Autodesk Fusion 360 part; units mm, degrees
(part 5 of 11)
  spline S16 degree 5 poles (47.8745, -68.1891) (47.8941, -68.2177) (47.934, -68.2742) (47.9958, -68.3575) (48.082, -68.4657) (48.1949, -68.5968) (48.3115, -68.7252) (48.4304, -68.8517) (48.5504, -68.9773) (48.6713, -69.1023) (48.793, -69.2265) (48.9159, -69.3498) (49.0402, -69.4719) (49.1663, -69.5925) (49.2941, -69.7117) (49.4235, -69.8295) (49.5542, -69.9462) (49.6861, -70.0619) (49.8189, -70.1767) (49.9526, -70.2907) (50.0871, -70.4039) (50.2227, -70.5162) (50.3592, -70.6276) (50.4968, -70.7381) (50.6354, -70.8476) (50.7749, -70.9562) (50.9154, -71.0639) (51.0567, -71.1709) (51.1988, -71.277) (51.3417, -71.3824) (51.4854, -71.487) (51.6299, -71.5908) (51.7751, -71.6938) (51.9212, -71.796) (52.068, -71.8975) (52.2156, -71.9982) (52.3638, -72.0981) (52.5129, -72.1974) (52.6626, -72.2958) (52.8129, -72.3936) (52.964, -72.4906) (53.1157, -72.587) (53.2681, -72.6826) (53.4212, -72.7775) (53.5749, -72.8717) (53.7292, -72.9652) (53.8842, -73.058) (54.0397, -73.1501) (54.1959, -73.2416) (54.3527, -73.3323) (54.51, -73.4224) (54.668, -73.5118) (54.8265, -73.6006) (54.9856, -73.6887) (55.1453, -73.7761) (55.3055, -73.8629) (55.4663, -73.949) (55.6276, -74.0344) (55.7895, -74.1192) (55.9519, -74.2034) (56.1148, -74.2869) (56.2783, -74.3698) (56.4422, -74.452) (56.6067, -74.5336) (56.7717, -74.6146) (56.9371, -74.695) (57.1031, -74.7747) (57.2696, -74.8537) (57.4365, -74.9322) (57.6039, -75.01) (57.7718, -75.0873) (57.9065, -75.1485) (58.0078, -75.1942) (58.0753, -75.2245) (58.1092, -75.2397) knots 0 0 0 0 0 0 0.01428571 0.02857143 0.04285714 0.05714286 0.07142857 0.08571429 0.1 0.11428571 0.12857143 0.14285714 0.15714286 0.17142857 0.18571429 0.2 0.21428571 0.22857143 0.24285714 0.25714286 0.27142857 0.28571429 0.3 0.31428571 0.32857143 0.34285714 0.35714286 0.37142857 0.38571429 0.4 0.41428571 0.42857143 0.44285714 0.45714286 0.47142857 0.48571429 0.5 0.51428571 0.52857143 0.54285714 0.55714286 0.57142857 0.58571429 0.6 0.61428571 0.62857143 0.64285714 0.65714286 0.67142857 0.68571429 0.7 0.71428571 0.72857143 0.74285714 0.75714286 0.77142857 0.78571429 0.8 0.81428571 0.82857143 0.84285714 0.85714286 0.87142857 0.88571429 0.9 0.91428571 0.92857143 0.94285714 0.95714286 0.97142857 0.98571429 1 1 1 1 1 1
  arc A38 (58.1092, -75.2397) -> (61.7381, -72.3457) centre (0.5538, 0.6546) ccw
  spline S17 degree 5 poles (57.1417, -60.7988) (57.1652, -60.8242) (57.2114, -60.8757) (57.2789, -60.9545) (57.3651, -61.0626) (57.4679, -61.2019) (57.5671, -61.3441) (57.664, -61.4881) (57.7597, -61.6331) (57.8547, -61.7788) (57.9487, -61.9251) (58.0416, -62.0723) (58.1329, -62.2207) (58.2225, -62.3705) (58.3102, -62.5216) (58.3963, -62.6739) (58.481, -62.8274) (58.5644, -62.9817) (58.6468, -63.1367) (58.7282, -63.2924) (58.8086, -63.4488) (58.8879, -63.6059) (58.9662, -63.7638) (59.0432, -63.9225) (59.1192, -64.082) (59.194, -64.2422) (59.2678, -64.4031) (59.3406, -64.5647) (59.4125, -64.7268) (59.4834, -64.8896) (59.5534, -65.053) (59.6224, -65.2169) (59.6905, -65.3815) (59.7577, -65.5466) (59.824, -65.7123) (59.8893, -65.8786) (59.9537, -66.0454) (60.0173, -66.2127) (60.08, -66.3806) (60.1419, -66.549) (60.2029, -66.7178) (60.263, -66.8872) (60.3223, -67.0571) (60.3808, -67.2274) (60.4384, -67.3982) (60.4952, -67.5695) (60.5512, -67.7412) (60.6064, -67.9133) (60.6608, -68.086) (60.7144, -68.259) (60.7673, -68.4325) (60.8193, -68.6064) (60.8705, -68.7807) (60.921, -68.9554) (60.9707, -69.1305) (61.0196, -69.306) (61.0678, -69.4819) (61.1152, -69.6582) (61.1619, -69.8349) (61.2078, -70.0119) (61.253, -70.1894) (61.2974, -70.3672) (61.3411, -70.5453) (61.3841, -70.7238) (61.4263, -70.9027) (61.4678, -71.0819) (61.5086, -71.2614) (61.5486, -71.4413) (61.588, -71.6215) (61.6266, -71.8021) (61.6645, -71.9829) (61.6943, -72.1279) (61.7163, -72.2367) (61.7308, -72.3094) (61.7381, -72.3457) knots 0 0 0 0 0 0 0.01428571 0.02857143 0.04285714 0.05714286 0.07142857 0.08571429 0.1 0.11428571 0.12857143 0.14285714 0.15714286 0.17142857 0.18571429 0.2 0.21428571 0.22857143 0.24285714 0.25714286 0.27142857 0.28571429 0.3 0.31428571 0.32857143 0.34285714 0.35714286 0.37142857 0.38571429 0.4 0.41428571 0.42857143 0.44285714 0.45714286 0.47142857 0.48571429 0.5 0.51428571 0.52857143 0.54285714 0.55714286 0.57142857 0.58571429 0.6 0.61428571 0.62857143 0.64285714 0.65714286 0.67142857 0.68571429 0.7 0.71428571 0.72857143 0.74285714 0.75714286 0.77142857 0.78571429 0.8 0.81428571 0.82857143 0.84285714 0.85714286 0.87142857 0.88571429 0.9 0.91428571 0.92857143 0.94285714 0.95714286 0.97142857 0.98571429 1 1 1 1 1 1
  line L17 (57.1417, -60.7988) -> (56.1297, -59.6994)
  arc A39 (56.1704, -58.5831) -> (56.1297, -59.6994) centre (56.7137, -59.1618) ccw
  arc A40 (56.1704, -58.5831) -> (59.7916, -54.9619) centre (0.5538, 0.6546) ccw
  arc A41 (60.9079, -54.9212) -> (59.7916, -54.9619) centre (60.3703, -55.5052) ccw
  line L18 (60.9079, -54.9212) -> (62.0072, -55.9332)
  spline S18 degree 5 poles (62.0072, -55.9332) (62.0327, -55.9567) (62.0842, -56.003) (62.163, -56.0704) (62.2711, -56.1566) (62.4104, -56.2594) (62.5526, -56.3586) (62.6966, -56.4555) (62.8416, -56.5513) (62.9873, -56.6462) (63.1336, -56.7402) (63.2808, -56.8331) (63.4292, -56.9245) (63.579, -57.014) (63.7301, -57.1018) (63.8824, -57.1878) (64.0358, -57.2725) (64.1901, -57.3559) (64.3452, -57.4383) (64.5009, -57.5197) (64.6573, -57.6001) (64.8144, -57.6795) (64.9723, -57.7577) (65.131, -57.8347) (65.2905, -57.9107) (65.4507, -57.9855) (65.6116, -58.0593) (65.7731, -58.1321) (65.9353, -58.204) (66.0981, -58.2749) (66.2614, -58.3449) (66.4254, -58.4139) (66.5899, -58.4821) (66.7551, -58.5492) (66.9208, -58.6155) (67.0871, -58.6808) (67.2539, -58.7453) (67.4212, -58.8088) (67.5891, -58.8715) (67.7575, -58.9334) (67.9263, -58.9944) (68.0957, -59.0545) (68.2655, -59.1138) (68.4359, -59.1723) (68.6067, -59.2299) (68.7779, -59.2868) (68.9497, -59.3428) (69.1218, -59.398) (69.2944, -59.4524) (69.4675, -59.506) (69.6409, -59.5588) (69.8148, -59.6108) (69.9891, -59.662) (70.1639, -59.7125) (70.339, -59.7622) (70.5145, -59.8112) (70.6904, -59.8593) (70.8667, -59.9067) (71.0434, -59.9534) (71.2204, -59.9993) (71.3978, -60.0445) (71.5756, -60.0889) (71.7538, -60.1326) (71.9323, -60.1756) (72.1112, -60.2178) (72.2904, -60.2593) (72.4699, -60.3001) (72.6498, -60.3402) (72.83, -60.3795) (73.0105, -60.4181) (73.1914, -60.4561) (73.3364, -60.4858) (73.4452, -60.5078) (73.5179, -60.5224) (73.5542, -60.5296) knots 0 0 0 0 0 0 0.01428571 0.02857143 0.04285714 0.05714286 0.07142857 0.08571429 0.1 0.11428571 0.12857143 0.14285714 0.15714286 0.17142857 0.18571429 0.2 0.21428571 0.22857143 0.24285714 0.25714286 0.27142857 0.28571429 0.3 0.31428571 0.32857143 0.34285714 0.35714286 0.37142857 0.38571429 0.4 0.41428571 0.42857143 0.44285714 0.45714286 0.47142857 0.48571429 0.5 0.51428571 0.52857143 0.54285714 0.55714286 0.57142857 0.58571429 0.6 0.61428571 0.62857143 0.64285714 0.65714286 0.67142857 0.68571429 0.7 0.71428571 0.72857143 0.74285714 0.75714286 0.77142857 0.78571429 0.8 0.81428571 0.82857143 0.84285714 0.85714286 0.87142857 0.88571429 0.9 0.91428571 0.92857143 0.94285714 0.95714286 0.97142857 0.98571429 1 1 1 1 1 1
  arc A42 (73.5542, -60.5296) -> (76.4482, -56.9007) centre (0.5538, 0.6546) ccw
  spline S19 degree 5 poles (69.3976, -46.666) (69.4262, -46.6856) (69.4827, -46.7255) (69.566, -46.7874) (69.6741, -46.8736) (69.8053, -46.9865) (69.9336, -47.103) (70.0602, -47.2219) (70.1858, -47.342) (70.3108, -47.4628) (70.435, -47.5846) (70.5583, -47.7074) (70.6804, -47.8317) (70.801, -47.9578) (70.9202, -48.0856) (71.038, -48.215) (71.1547, -48.3457) (71.2704, -48.4776) (71.3852, -48.6104) (71.4992, -48.7441) (71.6124, -48.8787) (71.7247, -49.0142) (71.8361, -49.1508) (71.9465, -49.2883) (72.0561, -49.4269) (72.1647, -49.5664) (72.2724, -49.7069) (72.3794, -49.8482) (72.4855, -49.9903) (72.5909, -50.1332) (72.6954, -50.2769) (72.7992, -50.4214) (72.9023, -50.5667) (73.0045, -50.7127) (73.106, -50.8595) (73.2067, -51.0071) (73.3066, -51.1554) (73.4058, -51.3044) (73.5043, -51.4541) (73.6021, -51.6045) (73.6991, -51.7555) (73.7954, -51.9073) (73.8911, -52.0596) (73.986, -52.2127) (74.0802, -52.3664) (74.1737, -52.5207) (74.2665, -52.6757) (74.3586, -52.8312) (74.45, -52.9874) (74.5408, -53.1442) (74.6309, -53.3016) (74.7203, -53.4595) (74.8091, -53.618) (74.8972, -53.7772) (74.9846, -53.9368) (75.0713, -54.097) (75.1575, -54.2578) (75.2429, -54.4191) (75.3277, -54.581) (75.4119, -54.7434) (75.4954, -54.9063) (75.5783, -55.0698) (75.6605, -55.2337) (75.7421, -55.3982) (75.8231, -55.5632) (75.9034, -55.7287) (75.9831, -55.8946) (76.0622, -56.0611) (76.1407, -56.228) (76.2185, -56.3954) (76.2957, -56.5633) (76.357, -56.698) (76.4027, -56.7993) (76.433, -56.8669) (76.4482, -56.9007) knots 0 0 0 0 0 0 0.01428571 0.02857143 0.04285714 0.05714286 0.07142857 0.08571429 0.1 0.11428571 0.12857143 0.14285714 0.15714286 0.17142857 0.18571429 0.2 0.21428571 0.22857143 0.24285714 0.25714286 0.27142857 0.28571429 0.3 0.31428571 0.32857143 0.34285714 0.35714286 0.37142857 0.38571429 0.4 0.41428571 0.42857143 0.44285714 0.45714286 0.47142857 0.48571429 0.5 0.51428571 0.52857143 0.54285714 0.55714286 0.57142857 0.58571429 0.6 0.61428571 0.62857143 0.64285714 0.65714286 0.67142857 0.68571429 0.7 0.71428571 0.72857143 0.74285714 0.75714286 0.77142857 0.78571429 0.8 0.81428571 0.82857143 0.84285714 0.85714286 0.87142857 0.88571429 0.9 0.91428571 0.92857143 0.94285714 0.95714286 0.97142857 0.98571429 1 1 1 1 1 1
  line L19 (69.3976, -46.666) -> (68.1663, -45.8194)
  arc A43 (67.9576, -44.7221) -> (68.1663, -45.8194) centre (68.616, -45.1653) ccw
  arc A44 (67.9576, -44.7221) -> (70.6822, -40.3858) centre (0.5538, 0.6546) ccw
  arc A45 (71.7614, -40.0978) -> (70.6822, -40.3858) centre (71.3673, -40.7867) ccw
  line L20 (71.7614, -40.0978) -> (73.0585, -40.8398)
  spline S20 degree 5 poles (73.0585, -40.8398) (73.0885, -40.857) (73.149, -40.8906) (73.2409, -40.9389) (73.3654, -40.9989) (73.5241, -41.0681) (73.6848, -41.1331) (73.8468, -41.1956) (74.0095, -41.2566) (74.1726, -41.3168) (74.3362, -41.3759) (74.5003, -41.4337) (74.6653, -41.4898) (74.8313, -41.5437) (74.9981, -41.5957) (75.1658, -41.6457) (75.3342, -41.6941) (75.5032, -41.7411) (75.6727, -41.7869) (75.8426, -41.8316) (76.013, -41.8752) (76.1838, -41.9176) (76.3552, -41.9587) (76.527, -41.9985) (76.6994, -42.0371) (76.8722, -42.0744) (77.0455, -42.1105) (77.2192, -42.1456) (77.3933, -42.1795) (77.5678, -42.2125) (77.7426, -42.2443) (77.9179, -42.2752) (78.0934, -42.305) (78.2694, -42.3337) (78.4457, -42.3614) (78.6223, -42.3881) (78.7993, -42.4138) (78.9766, -42.4386) (79.1542, -42.4623) (79.3321, -42.4852) (79.5103, -42.5071) (79.6888, -42.528) (79.8676, -42.548) (80.0467, -42.5671) (80.226, -42.5853) (80.4056, -42.6026) (80.5855, -42.619) (80.7656, -42.6345) (80.946, -42.6491) (81.1267, -42.6629) (81.3075, -42.6758) (81.4886, -42.6878) (81.67, -42.699) (81.8515, -42.7093) (82.0333, -42.7188) (82.2153, -42.7274) (82.3976, -42.7353) (82.58, -42.7423) (82.7626, -42.7484) (82.9454, -42.7538) (83.1285, -42.7584) (83.3117, -42.7621) (83.4951, -42.7651) (83.6787, -42.7672) (83.8625, -42.7686) (84.0464, -42.7692) (84.2305, -42.769) (84.4148, -42.768) (84.5993, -42.7663) (84.7839, -42.7638) (84.9686, -42.7605) (85.1166, -42.7573) (85.2276, -42.7545) (85.3017, -42.7525) (85.3387, -42.7515) knots 0 0 0 0 0 0 0.01428571 0.02857143 0.04285714 0.05714286 0.07142857 0.08571429 0.1 0.11428571 0.12857143 0.14285714 0.15714286 0.17142857 0.18571429 0.2 0.21428571 0.22857143 0.24285714 0.25714286 0.27142857 0.28571429 0.3 0.31428571 0.32857143 0.34285714 0.35714286 0.37142857 0.38571429 0.4 0.41428571 0.42857143 0.44285714 0.45714286 0.47142857 0.48571429 0.5 0.51428571 0.52857143 0.54285714 0.55714286 0.57142857 0.58571429 0.6 0.61428571 0.62857143 0.64285714 0.65714286 0.67142857 0.68571429 0.7 0.71428571 0.72857143 0.74285714 0.75714286 0.77142857 0.78571429 0.8 0.81428571 0.82857143 0.84285714 0.85714286 0.87142857 0.88571429 0.9 0.91428571 0.92857143 0.94285714 0.95714286 0.97142857 0.98571429 1 1 1 1 1 1
  arc A46 (85.3387, -42.7515) -> (87.3526, -38.5696) centre (0.5538, 0.6546) ccw
  spline S21 degree 5 poles (78.2014, -30.1604) (78.2336, -30.1732) (78.2976, -30.1995) (78.3926, -30.2412) (78.5172, -30.3012) (78.6702, -30.3821) (78.8212, -30.4672) (78.9711, -30.5549) (79.1202, -30.644) (79.269, -30.7341) (79.4172, -30.8251) (79.5647, -30.9174) (79.7114, -31.0115) (79.8571, -31.1075) (80.0017, -31.2056) (80.1454, -31.3055) (80.2882, -31.407) (80.4303, -31.5098) (80.5718, -31.6138) (80.7127, -31.7187) (80.853, -31.8248) (80.9927, -31.9319) (81.1316, -32.0402) (81.2699, -32.1498) (81.4075, -32.2605) (81.5445, -32.3724) (81.6808, -32.4853) (81.8165, -32.5993) (81.9516, -32.7142) (82.0861, -32.8301) (82.22, -32.9469) (82.3534, -33.0647) (82.4862, -33.1834) (82.6183, -33.303) (82.7499, -33.4236) (82.8809, -33.545) (83.0114, -33.6674) (83.1413, -33.7906) (83.2706, -33.9146) (83.3993, -34.0395) (83.5276, -34.1651) (83.6552, -34.2916) (83.7824, -34.4189) (83.909, -34.547) (84.035, -34.6759) (84.1605, -34.8055) (84.2855, -34.936) (84.4099, -35.0671) (84.5338, -35.199) (84.6572, -35.3317) (84.78, -35.4651) (84.9023, -35.5992) (85.0241, -35.734) (85.1454, -35.8695) (85.2662, -36.0057) (85.3864, -36.1426) (85.5062, -36.2802) (85.6254, -36.4185) (85.7441, -36.5574) (85.8623, -36.697) (85.9799, -36.8372) (86.0971, -36.9781) (86.2138, -37.1197) (86.3299, -37.2619) (86.4456, -37.4047) (86.5607, -37.5482) (86.6754, -37.6922) (86.7895, -37.8369) (86.9032, -37.9822) (87.0163, -38.1281) (87.1289, -38.2746) (87.2186, -38.3923) (87.2857, -38.4808) (87.3303, -38.54) (87.3526, -38.5696) knots 0 0 0 0 0 0 0.01428571 0.02857143 0.04285714 0.05714286 0.07142857 0.08571429 0.1 0.11428571 0.12857143 0.14285714 0.15714286 0.17142857 0.18571429 0.2 0.21428571 0.22857143 0.24285714 0.25714286 0.27142857 0.28571429 0.3 0.31428571 0.32857143 0.34285714 0.35714286 0.37142857 0.38571429 0.4 0.41428571 0.42857143 0.44285714 0.45714286 0.47142857 0.48571429 0.5 0.51428571 0.52857143 0.54285714 0.55714286 0.57142857 0.58571429 0.6 0.61428571 0.62857143 0.64285714 0.65714286 0.67142857 0.68571429 0.7 0.71428571 0.72857143 0.74285714 0.75714286 0.77142857 0.78571429 0.8 0.81428571 0.82857143 0.84285714 0.85714286 0.87142857 0.88571429 0.9 0.91428571 0.92857143 0.94285714 0.95714286 0.97142857 0.98571429 1 1 1 1 1 1
  line L21 (78.2014, -30.1604) -> (76.8126, -29.609)
  arc A47 (76.3649, -28.5856) -> (76.8126, -29.609) centre (77.1055, -28.8713) ccw
  arc A48 (76.3649, -28.5856) -> (78.0563, -23.7518) centre (0.5538, 0.6546) ccw
  arc A49 (79.0444, -23.2308) -> (78.0563, -23.7518) centre (78.8134, -23.9902) ccw
  line L22 (79.0444, -23.2308) -> (80.474, -23.6657)
  spline S22 degree 5 poles (80.474, -23.6657) (80.5071, -23.6757) (80.5736, -23.6951) (80.6739, -23.7216) (80.8087, -23.7524) (80.9787, -23.7846) (81.1499, -23.8122) (81.3217, -23.8371) (81.4939, -23.8604) (81.6663, -23.8828) (81.839, -23.904) (82.0119, -23.9238) (82.1852, -23.9417) (82.359, -23.9575) (82.5332, -23.9709) (82.7078, -23.9824) (82.8828, -23.9921) (83.058, -24.0003) (83.2334, -24.0073) (83.409, -24.0131) (83.5848, -24.0177) (83.7608, -24.021) (83.937, -24.0229) (84.1134, -24.0235) (84.2901, -24.0227) (84.4669, -24.0206) (84.6439, -24.0173) (84.821, -24.0128) (84.9983, -24.0072) (85.1757, -24.0005) (85.3533, -23.9926) (85.531, -23.9837) (85.7088, -23.9737) (85.8867, -23.9626) (86.0647, -23.9504) (86.2429, -23.9371) (86.4212, -23.9228) (86.5995, -23.9074) (86.7779, -23.8911) (86.9565, -23.8738) (87.1351, -23.8554) (87.3138, -23.8361) (87.4925, -23.8159) (87.6714, -23.7947) (87.8503, -23.7725) (88.0292, -23.7494) (88.2082, -23.7253) (88.3873, -23.7003) (88.5664, -23.6745) (88.7456, -23.6477) (88.9248, -23.62) (89.104, -23.5914) (89.2833, -23.562) (89.4626, -23.5316) (89.642, -23.5004) (89.8213, -23.4684) (90.0007, -23.4355) (90.1801, -23.4017) (90.3596, -23.3671) (90.539, -23.3316) (90.7185, -23.2953) (90.8979, -23.2582) (91.0774, -23.2203) (91.2568, -23.1815) (91.4363, -23.142) (91.6158, -23.1016) (91.7952, -23.0605) (91.9747, -23.0185) (92.1541, -22.9758) (92.3336, -22.9322) (92.513, -22.8879) (92.6565, -22.8519) (92.7641, -22.8245) (92.8359, -22.806) (92.8717, -22.7968) knots 0 0 0 0 0 0 0.01428571 0.02857143 0.04285714 0.05714286 0.07142857 0.08571429 0.1 0.11428571 0.12857143 0.14285714 0.15714286 0.17142857 0.18571429 0.2 0.21428571 0.22857143 0.24285714 0.25714286 0.27142857 0.28571429 0.3 0.31428571 0.32857143 0.34285714 0.35714286 0.37142857 0.38571429 0.4 0.41428571 0.42857143 0.44285714 0.45714286 0.47142857 0.48571429 0.5 0.51428571 0.52857143 0.54285714 0.55714286 0.57142857 0.58571429 0.6 0.61428571 0.62857143 0.64285714 0.65714286 0.67142857 0.68571429 0.7 0.71428571 0.72857143 0.74285714 0.75714286 0.77142857 0.78571429 0.8 0.81428571 0.82857143 0.84285714 0.85714286 0.87142857 0.88571429 0.9 0.91428571 0.92857143 0.94285714 0.95714286 0.97142857 0.98571429 1 1 1 1 1 1
  arc A50 (92.8717, -22.7968) -> (93.9046, -18.2716) centre (0.5538, 0.6546) ccw
  spline S23 degree 5 poles (83.1116, -12.1096) (83.1458, -12.1149) (83.2141, -12.1263) (83.316, -12.1459) (83.4508, -12.1766) (83.618, -12.2214) (83.7842, -12.2708) (83.9497, -12.3229) (84.115, -12.3766) (84.28, -12.4313) (84.4448, -12.4871) (84.6092, -12.5442) (84.7731, -12.6033) (84.9365, -12.6646) (85.0993, -12.728) (85.2616, -12.7934) (85.4235, -12.8606) (85.5849, -12.9292) (85.746, -12.999) (85.9067, -13.07) (86.0671, -13.1422) (86.2271, -13.2156) (86.3867, -13.2903) (86.5459, -13.3663) (86.7047, -13.4436) (86.8631, -13.5222) (87.0211, -13.602) (87.1788, -13.6829) (87.336, -13.7649) (87.493, -13.8479) (87.6495, -13.932) (87.8058, -14.0172) (87.9616, -14.1033) (88.1171, -14.1906) (88.2722, -14.2788) (88.427, -14.3681) (88.5814, -14.4583) (88.7354, -14.5495) (88.8891, -14.6417) (89.0424, -14.7347) (89.1954, -14.8287) (89.348, -14.9236) (89.5003, -15.0195) (89.6522, -15.1162) (89.8037, -15.2138) (89.9549, -15.3123) (90.1058, -15.4116) (90.2563, -15.5118) (90.4064, -15.6128) (90.5562, -15.7147) (90.7057, -15.8174) (90.8548, -15.9209) (91.0035, -16.0252) (91.1519, -16.1304) (91.3, -16.2363) (91.4477, -16.343) (91.595, -16.4505) (91.742, -16.5588) (91.8886, -16.6678) (92.0349, -16.7776) (92.1809, -16.8881) (92.3264, -16.9994) (92.4717, -17.1115) (92.6166, -17.2243) (92.7611, -17.3378) (92.9053, -17.452) (93.0491, -17.5669) (93.1926, -17.6826) (93.3357, -17.799) (93.4785, -17.916) (93.6209, -18.0338) (93.7345, -18.1286) (93.8196, -18.2) (93.8763, -18.2477) (93.9046, -18.2716) knots 0 0 0 0 0 0 0.01428571 0.02857143 0.04285714 0.05714286 0.07142857 0.08571429 0.1 0.11428571 0.12857143 0.14285714 0.15714286 0.17142857 0.18571429 0.2 0.21428571 0.22857143 0.24285714 0.25714286 0.27142857 0.28571429 0.3 0.31428571 0.32857143 0.34285714 0.35714286 0.37142857 0.38571429 0.4 0.41428571 0.42857143 0.44285714 0.45714286 0.47142857 0.48571429 0.5 0.51428571 0.52857143 0.54285714 0.55714286 0.57142857 0.58571429 0.6 0.61428571 0.62857143 0.64285714 0.65714286 0.67142857 0.68571429 0.7 0.71428571 0.72857143 0.74285714 0.75714286 0.77142857 0.78571429 0.8 0.81428571 0.82857143 0.84285714 0.85714286 0.87142857 0.88571429 0.9 0.91428571 0.92857143 0.94285714 0.95714286 0.97142857 0.98571429 1 1 1 1 1 1
  line L23 (83.1116, -12.1096) -> (81.6349, -11.8811)
  arc A51 (80.9707, -10.983) -> (81.6349, -11.8811) centre (81.7563, -11.0966) ccw
  arc A52 (80.9707, -10.983) -> (81.5441, -5.894) centre (0.5538, 0.6546) ccw
  arc A53 (82.3915, -5.1662) -> (81.5441, -5.894) centre (82.3353, -5.958) ccw
  line L24 (82.3915, -5.1662) -> (83.882, -5.272)
  spline S24 degree 5 poles (83.882, -5.272) (83.9166, -5.2744) (83.9856, -5.2785) (84.0893, -5.2821) (84.2276, -5.2821) (84.4006, -5.2756) (84.5736, -5.2645) (84.7466, -5.2505) (84.9197, -5.2349) (85.0927, -5.2183) (85.2658, -5.2006) (85.4388, -5.1815) (85.6118, -5.1604) (85.7847, -5.137) (85.9575, -5.1114) (86.1303, -5.0837) (86.303, -5.0542) (86.4757, -5.0233) (86.6483, -4.991) (86.8208, -4.9576) (86.9932, -4.9229) (87.1655, -4.887) (87.3377, -4.8497) (87.5098, -4.811) (87.6819, -4.7709) (87.8538, -4.7296) (88.0256, -4.6869) (88.1973, -4.6431) (88.3689, -4.5982) (88.5404, -4.5522) (88.7117, -4.505) (88.883, -4.4568) (89.0541, -4.4075) (89.2251, -4.357) (89.3959, -4.3055) (89.5667, -4.2529) (89.7373, -4.1993) (89.9077, -4.1446) (90.0781, -4.089) (90.2483, -4.0324) (90.4183, -3.9748) (90.5882, -3.9162) (90.758, -3.8567) (90.9276, -3.7962) (91.0971, -3.7348) (91.2664, -3.6724) (91.4356, -3.6091) (91.6046, -3.5449) (91.7735, -3.4798) (91.9422, -3.4139) (92.1108, -3.347) (92.2792, -3.2793) (92.4474, -3.2106) (92.6155, -3.1412) (92.7834, -3.0708) (92.9511, -2.9997) (93.1187, -2.9277) (93.2861, -2.8548) (93.4533, -2.7811) (93.6203, -2.7067) (93.7872, -2.6313) (93.9539, -2.5552) (94.1204, -2.4783) (94.2868, -2.4006) (94.453, -2.3221) (94.6189, -2.2428) (94.7847, -2.1628) (94.9504, -2.0819) (95.1158, -2.0003) (95.281, -1.918) (95.4461, -1.8348) (95.578, -1.7677) (95.6768, -1.7171) (95.7426, -1.6831) (95.7756, -1.6661) knots 0 0 0 0 0 0 0.01428571 0.02857143 0.04285714 0.05714286 0.07142857 0.08571429 0.1 0.11428571 0.12857143 0.14285714 0.15714286 0.17142857 0.18571429 0.2 0.21428571 0.22857143 0.24285714 0.25714286 0.27142857 0.28571429 0.3 0.31428571 0.32857143 0.34285714 0.35714286 0.37142857 0.38571429 0.4 0.41428571 0.42857143 0.44285714 0.45714286 0.47142857 0.48571429 0.5 0.51428571 0.52857143 0.54285714 0.55714286 0.57142857 0.58571429 0.6 0.61428571 0.62857143 0.64285714 0.65714286 0.67142857 0.68571429 0.7 0.71428571 0.72857143 0.74285714 0.75714286 0.77142857 0.78571429 0.8 0.81428571 0.82857143 0.84285714 0.85714286 0.87142857 0.88571429 0.9 0.91428571 0.92857143 0.94285714 0.95714286 0.97142857 0.98571429 1 1 1 1 1 1
  arc A54 (95.7756, -1.6661) -> (95.7756, 2.9754) centre (0.5538, 0.6546) ccw
  spline S25 degree 5 poles (83.882, 6.5813) (83.9166, 6.5837) (83.9856, 6.5878) (84.0893, 6.5914) (84.2276, 6.5914) (84.4006, 6.5849) (84.5736, 6.5738) (84.7466, 6.5598) (84.9197, 6.5442) (85.0927, 6.5276) (85.2658, 6.5099) (85.4388, 6.4908) (85.6118, 6.4697) (85.7847, 6.4463) (85.9575, 6.4207) (86.1303, 6.393) (86.303, 6.3635) (86.4757, 6.3326) (86.6483, 6.3003) (86.8208, 6.2669) (86.9932, 6.2322) (87.1655, 6.1963) (87.3377, 6.159) (87.5098, 6.1203) (87.6819, 6.0802) (87.8538, 6.0388) (88.0256, 5.9962) (88.1973, 5.9524) (88.3689, 5.9075) (88.5404, 5.8615) (88.7117, 5.8143) (88.883, 5.7661) (89.0541, 5.7167) (89.2251, 5.6663) (89.3959, 5.6148) (89.5667, 5.5622) (89.7373, 5.5086) (89.9077, 5.4539) (90.0781, 5.3983) (90.2483, 5.3417) (90.4183, 5.2841) (90.5882, 5.2255) (90.758, 5.166) (90.9276, 5.1055) (91.0971, 5.044) (91.2664, 4.9817) (91.4356, 4.9184) (91.6046, 4.8542) (91.7735, 4.7891) (91.9422, 4.7231) (92.1108, 4.6563) (92.2792, 4.5885) (92.4474, 4.5199) (92.6155, 4.4504) (92.7834, 4.3801) (92.9511, 4.3089) (93.1187, 4.2369) (93.2861, 4.1641) (93.4533, 4.0904) (93.6203, 4.0159) (93.7872, 3.9406) (93.9539, 3.8645) (94.1204, 3.7876) (94.2868, 3.7099) (94.453, 3.6314) (94.6189, 3.5521) (94.7847, 3.472) (94.9504, 3.3912) (95.1158, 3.3096) (95.281, 3.2272) (95.4461, 3.1441) (95.578, 3.077) (95.6768, 3.0263) (95.7426, 2.9924) (95.7756, 2.9754) knots 0 0 0 0 0 0 0.01428571 0.02857143 0.04285714 0.05714286 0.07142857 0.08571429 0.1 0.11428571 0.12857143 0.14285714 0.15714286 0.17142857 0.18571429 0.2 0.21428571 0.22857143 0.24285714 0.25714286 0.27142857 0.28571429 0.3 0.31428571 0.32857143 0.34285714 0.35714286 0.37142857 0.38571429 0.4 0.41428571 0.42857143 0.44285714 0.45714286 0.47142857 0.48571429 0.5 0.51428571 0.52857143 0.54285714 0.55714286 0.57142857 0.58571429 0.6 0.61428571 0.62857143 0.64285714 0.65714286 0.67142857 0.68571429 0.7 0.71428571 0.72857143 0.74285714 0.75714286 0.77142857 0.78571429 0.8 0.81428571 0.82857143 0.84285714 0.85714286 0.87142857 0.88571429 0.9 0.91428571 0.92857143 0.94285714 0.95714286 0.97142857 0.98571429 1 1 1 1 1 1
  line L25 (83.882, 6.5813) -> (82.3915, 6.4755)
  arc A55 (81.5441, 7.2033) -> (82.3915, 6.4755) centre (82.3353, 7.2672) ccw
  arc A56 (81.5441, 7.2033) -> (80.9707, 12.2922) centre (0.5538, 0.6546) ccw
  arc A57 (81.6349, 13.1903) -> (80.9707, 12.2922) centre (81.7563, 12.4059) ccw
  line L26 (81.6349, 13.1903) -> (83.1116, 13.4189)
  spline S26 degree 5 poles (83.1116, 13.4189) (83.1458, 13.4242) (83.2141, 13.4356) (83.316, 13.4551) (83.4508, 13.4859) (83.618, 13.5307) (83.7842, 13.5801) (83.9497, 13.6322) (84.115, 13.6859) (84.28, 13.7406) (84.4448, 13.7963) (84.6092, 13.8535) (84.7731, 13.9126) (84.9365, 13.9738) (85.0993, 14.0373) (85.2616, 14.1027) (85.4235, 14.1699) (85.5849, 14.2385) (85.746, 14.3083) (85.9067, 14.3793) (86.0671, 14.4515) (86.2271, 14.5248) (86.3867, 14.5995) (86.5459, 14.6756) (86.7047, 14.7529) (86.8631, 14.8315) (87.0211, 14.9113) (87.1788, 14.9922) (87.336, 15.0742) (87.493, 15.1572) (87.6495, 15.2413) (87.8058, 15.3264) (87.9616, 15.4126) (88.1171, 15.4998) (88.2722, 15.5881) (88.427, 15.6774) (88.5814, 15.7676) (88.7354, 15.8588) (88.8891, 15.9509) (89.0424, 16.044) (89.1954, 16.138) (89.348, 16.2329) (89.5003, 16.3287) (89.6522, 16.4255) (89.8037, 16.5231) (89.9549, 16.6215) (90.1058, 16.7209) (90.2563, 16.8211) (90.4064, 16.9221) (90.5562, 17.024) (90.7057, 17.1267) (90.8548, 17.2302) (91.0035, 17.3345) (91.1519, 17.4396) (91.3, 17.5456) (91.4477, 17.6523) (91.595, 17.7598) (91.742, 17.868) (91.8886, 17.9771) (92.0349, 18.0869) (92.1809, 18.1974) (92.3264, 18.3087) (92.4717, 18.4208) (92.6166, 18.5335) (92.7611, 18.647) (92.9053, 18.7613) (93.0491, 18.8762) (93.1926, 18.9919) (93.3357, 19.1082) (93.4785, 19.2253) (93.6209, 19.3431) (93.7345, 19.4379) (93.8196, 19.5092) (93.8763, 19.557) (93.9046, 19.5809) knots 0 0 0 0 0 0 0.01428571 0.02857143 0.04285714 0.05714286 0.07142857 0.08571429 0.1 0.11428571 0.12857143 0.14285714 0.15714286 0.17142857 0.18571429 0.2 0.21428571 0.22857143 0.24285714 0.25714286 0.27142857 0.28571429 0.3 0.31428571 0.32857143 0.34285714 0.35714286 0.37142857 0.38571429 0.4 0.41428571 0.42857143 0.44285714 0.45714286 0.47142857 0.48571429 0.5 0.51428571 0.52857143 0.54285714 0.55714286 0.57142857 0.58571429 0.6 0.61428571 0.62857143 0.64285714 0.65714286 0.67142857 0.68571429 0.7 0.71428571 0.72857143 0.74285714 0.75714286 0.77142857 0.78571429 0.8 0.81428571 0.82857143 0.84285714 0.85714286 0.87142857 0.88571429 0.9 0.91428571 0.92857143 0.94285714 0.95714286 0.97142857 0.98571429 1 1 1 1 1 1
  arc A58 (93.9046, 19.5809) -> (92.8717, 24.1061) centre (0.5538, 0.6546) ccw
  spline S27 degree 5 poles (80.474, 24.9749) (80.5071, 24.985) (80.5736, 25.0043) (80.6739, 25.0309) (80.8087, 25.0617) (80.9787, 25.0939) (81.1499, 25.1215) (81.3217, 25.1464) (81.4939, 25.1697) (81.6663, 25.192) (81.839, 25.2133) (82.0119, 25.2331) (82.1852, 25.251) (82.359, 25.2667) (82.5332, 25.2802) (82.7078, 25.2917) (82.8828, 25.3014) (83.058, 25.3096) (83.2334, 25.3166) (83.409, 25.3224) (83.5848, 25.3269) (83.7608, 25.3302) (83.937, 25.3322) (84.1134, 25.3328) (84.2901, 25.332) (84.4669, 25.3299) (84.6439, 25.3266) (84.821, 25.3221) (84.9983, 25.3165) (85.1757, 25.3097) (85.3533, 25.3019) (85.531, 25.293) (85.7088, 25.283) (85.8867, 25.2718) (86.0647, 25.2596) (86.2429, 25.2464) (86.4212, 25.232) (86.5995, 25.2167) (86.7779, 25.2004) (86.9565, 25.183) (87.1351, 25.1647) (87.3138, 25.1454) (87.4925, 25.1252) (87.6714, 25.1039) (87.8503, 25.0818) (88.0292, 25.0586) (88.2082, 25.0346) (88.3873, 25.0096) (88.5664, 24.9837) (88.7456, 24.957) (88.9248, 24.9293) (89.104, 24.9007) (89.2833, 24.8712) (89.4626, 24.8409) (89.642, 24.8097) (89.8213, 24.7777) (90.0007, 24.7447) (90.1801, 24.711) (90.3596, 24.6763) (90.539, 24.6409) (90.7185, 24.6046) (90.8979, 24.5675) (91.0774, 24.5296) (91.2568, 24.4908) (91.4363, 24.4513) (91.6158, 24.4109) (91.7952, 24.3697) (91.9747, 24.3278) (92.1541, 24.2851) (92.3336, 24.2415) (92.513, 24.1972) (92.6565, 24.1611) (92.7641, 24.1337) (92.8359, 24.1153) (92.8717, 24.1061) knots 0 0 0 0 0 0 0.01428571 0.02857143 0.04285714 0.05714286 0.07142857 0.08571429 0.1 0.11428571 0.12857143 0.14285714 0.15714286 0.17142857 0.18571429 0.2 0.21428571 0.22857143 0.24285714 0.25714286 0.27142857 0.28571429 0.3 0.31428571 0.32857143 0.34285714 0.35714286 0.37142857 0.38571429 0.4 0.41428571 0.42857143 0.44285714 0.45714286 0.47142857 0.48571429 0.5 0.51428571 0.52857143 0.54285714 0.55714286 0.57142857 0.58571429 0.6 0.61428571 0.62857143 0.64285714 0.65714286 0.67142857 0.68571429 0.7 0.71428571 0.72857143 0.74285714 0.75714286 0.77142857 0.78571429 0.8 0.81428571 0.82857143 0.84285714 0.85714286 0.87142857 0.88571429 0.9 0.91428571 0.92857143 0.94285714 0.95714286 0.97142857 0.98571429 1 1 1 1 1 1
  line L27 (80.474, 24.9749) -> (79.0444, 24.5401)
  arc A59 (78.0563, 25.0611) -> (79.0444, 24.5401) centre (78.8134, 25.2995) ccw
  arc A60 (78.0563, 25.0611) -> (76.3649, 29.8949) centre (0.5538, 0.6546) ccw
  arc A61 (76.8126, 30.9183) -> (76.3649, 29.8949) centre (77.1055, 30.1805) ccw
  line L28 (76.8126, 30.9183) -> (78.2014, 31.4697)
  spline S28 degree 5 poles (78.2014, 31.4697) (78.2336, 31.4825) (78.2976, 31.5088) (78.3926, 31.5505) (78.5172, 31.6105) (78.6702, 31.6914) (78.8212, 31.7765) (78.9711, 31.8642) (79.1202, 31.9533) (79.269, 32.0433) (79.4172, 32.1344) (79.5647, 32.2267) (79.7114, 32.3207) (79.8571, 32.4168) (80.0017, 32.5149) (80.1454, 32.6148) (80.2882, 32.7163) (80.4303, 32.8191) (80.5718, 32.923) (80.7127, 33.028) (80.853, 33.134) (80.9927, 33.2412) (81.1316, 33.3495) (81.2699, 33.4591) (81.4075, 33.5698) (81.5445, 33.6817) (81.6808, 33.7946) (81.8165, 33.9086) (81.9516, 34.0235) (82.0861, 34.1394) (82.22, 34.2562) (82.3534, 34.374) (82.4862, 34.4927) (82.6183, 34.6123) (82.7499, 34.7329) (82.8809, 34.8543) (83.0114, 34.9766) (83.1413, 35.0998) (83.2706, 35.2239) (83.3993, 35.3487) (83.5276, 35.4744) (83.6552, 35.6009) (83.7824, 35.7282) (83.909, 35.8563) (84.035, 35.9852) (84.1605, 36.1148) (84.2855, 36.2452) (84.4099, 36.3764) (84.5338, 36.5083) (84.6572, 36.641) (84.78, 36.7743) (84.9023, 36.9084) (85.0241, 37.0433) (85.1454, 37.1788) (85.2662, 37.315) (85.3864, 37.4519) (85.5062, 37.5895) (85.6254, 37.7277) (85.7441, 37.8667) (85.8623, 38.0063) (85.9799, 38.1465) (86.0971, 38.2874) (86.2138, 38.429) (86.3299, 38.5712) (86.4456, 38.714) (86.5607, 38.8574) (86.6754, 39.0015) (86.7895, 39.1462) (86.9032, 39.2915) (87.0163, 39.4374) (87.1289, 39.5839) (87.2186, 39.7016) (87.2857, 39.7901) (87.3303, 39.8493) (87.3526, 39.8789) knots 0 0 0 0 0 0 0.01428571 0.02857143 0.04285714 0.05714286 0.07142857 0.08571429 0.1 0.11428571 0.12857143 0.14285714 0.15714286 0.17142857 0.18571429 0.2 0.21428571 0.22857143 0.24285714 0.25714286 0.27142857 0.28571429 0.3 0.31428571 0.32857143 0.34285714 0.35714286 0.37142857 0.38571429 0.4 0.41428571 0.42857143 0.44285714 0.45714286 0.47142857 0.48571429 0.5 0.51428571 0.52857143 0.54285714 0.55714286 0.57142857 0.58571429 0.6 0.61428571 0.62857143 0.64285714 0.65714286 0.67142857 0.68571429 0.7 0.71428571 0.72857143 0.74285714 0.75714286 0.77142857 0.78571429 0.8 0.81428571 0.82857143 0.84285714 0.85714286 0.87142857 0.88571429 0.9 0.91428571 0.92857143 0.94285714 0.95714286 0.97142857 0.98571429 1 1 1 1 1 1
  arc A62 (87.3526, 39.8789) -> (85.3387, 44.0607) centre (0.5538, 0.6546) ccw
  spline S29 degree 5 poles (73.0585, 42.1491) (73.0885, 42.1663) (73.149, 42.1999) (73.2409, 42.2481) (73.3654, 42.3082) (73.5241, 42.3774) (73.6848, 42.4424) (73.8468, 42.5049) (74.0095, 42.5659) (74.1726, 42.6261) (74.3362, 42.6852) (74.5003, 42.743) (74.6653, 42.799) (74.8313, 42.853) (74.9981, 42.9049) (75.1658, 42.955) (75.3342, 43.0033) (75.5032, 43.0504) (75.6727, 43.0962) (75.8426, 43.1409) (76.013, 43.1845) (76.1838, 43.2269) (76.3552, 43.268) (76.527, 43.3078) (76.6994, 43.3463) (76.8722, 43.3837) (77.0455, 43.4198) (77.2192, 43.4548) (77.3933, 43.4888) (77.5678, 43.5217) (77.7426, 43.5536) (77.9179, 43.5844) (78.0934, 43.6142) (78.2694, 43.643) (78.4457, 43.6707) (78.6223, 43.6974) (78.7993, 43.7231) (78.9766, 43.7478) (79.1542, 43.7716) (79.3321, 43.7945) (79.5103, 43.8163) (79.6888, 43.8373) (79.8676, 43.8573) (80.0467, 43.8764) (80.226, 43.8946) (80.4056, 43.9119) (80.5855, 43.9283) (80.7656, 43.9438) (80.946, 43.9584) (81.1267, 43.9722) (81.3075, 43.985) (81.4886, 43.9971) (81.67, 44.0083) (81.8515, 44.0186) (82.0333, 44.0281) (82.2153, 44.0367) (82.3976, 44.0445) (82.58, 44.0515) (82.7626, 44.0577) (82.9454, 44.0631) (83.1285, 44.0677) (83.3117, 44.0714) (83.4951, 44.0744) (83.6787, 44.0765) (83.8625, 44.0779) (84.0464, 44.0785) (84.2305, 44.0783) (84.4148, 44.0773) (84.5993, 44.0756) (84.7839, 44.0731) (84.9686, 44.0698) (85.1166, 44.0665) (85.2276, 44.0638) (85.3017, 44.0618) (85.3387, 44.0607) knots 0 0 0 0 0 0 0.01428571 0.02857143 0.04285714 0.05714286 0.07142857 0.08571429 0.1 0.11428571 0.12857143 0.14285714 0.15714286 0.17142857 0.18571429 0.2 0.21428571 0.22857143 0.24285714 0.25714286 0.27142857 0.28571429 0.3 0.31428571 0.32857143 0.34285714 0.35714286 0.37142857 0.38571429 0.4 0.41428571 0.42857143 0.44285714 0.45714286 0.47142857 0.48571429 0.5 0.51428571 0.52857143 0.54285714 0.55714286 0.57142857 0.58571429 0.6 0.61428571 0.62857143 0.64285714 0.65714286 0.67142857 0.68571429 0.7 0.71428571 0.72857143 0.74285714 0.75714286 0.77142857 0.78571429 0.8 0.81428571 0.82857143 0.84285714 0.85714286 0.87142857 0.88571429 0.9 0.91428571 0.92857143 0.94285714 0.95714286 0.97142857 0.98571429 1 1 1 1 1 1
  line L29 (73.0585, 42.1491) -> (71.7614, 41.4071)
  arc A63 (70.6822, 41.6951) -> (71.7614, 41.4071) centre (71.3673, 42.096) ccw
  arc A64 (70.6822, 41.6951) -> (67.9576, 46.0313) centre (0.5538, 0.6546) ccw
  arc A65 (68.1663, 47.1287) -> (67.9576, 46.0313) centre (68.616, 46.4746) ccw
  line L30 (68.1663, 47.1287) -> (69.3976, 47.9753)
  spline S30 degree 5 poles (69.3976, 47.9753) (69.4262, 47.9949) (69.4827, 48.0348) (69.566, 48.0966) (69.6741, 48.1828) (69.8053, 48.2957) (69.9336, 48.4123) (70.0602, 48.5312) (70.1858, 48.6512) (70.3108, 48.7721) (70.435, 48.8938) (70.5583, 49.0167) (70.6804, 49.141) (70.801, 49.2671) (70.9202, 49.3949) (71.038, 49.5243) (71.1547, 49.655) (71.2704, 49.7869) (71.3852, 49.9197) (71.4992, 50.0534) (71.6124, 50.1879) (71.7247, 50.3235) (71.8361, 50.46) (71.9465, 50.5976) (72.0561, 50.7362) (72.1647, 50.8757) (72.2724, 51.0162) (72.3794, 51.1575) (72.4855, 51.2996) (72.5909, 51.4425) (72.6954, 51.5862) (72.7992, 51.7307) (72.9023, 51.8759) (73.0045, 52.022) (73.106, 52.1688) (73.2067, 52.3164) (73.3066, 52.4646) (73.4058, 52.6136) (73.5043, 52.7633) (73.6021, 52.9137) (73.6991, 53.0648) (73.7954, 53.2165) (73.8911, 53.3689) (73.986, 53.522) (74.0802, 53.6757) (74.1737, 53.83) (74.2665, 53.9849) (74.3586, 54.1405) (74.45, 54.2967) (74.5408, 54.4535) (74.6309, 54.6108) (74.7203, 54.7688) (74.8091, 54.9273) (74.8972, 55.0864) (74.9846, 55.2461) (75.0713, 55.4063) (75.1575, 55.5671) (75.2429, 55.7284) (75.3277, 55.8903) (75.4119, 56.0527) (75.4954, 56.2156) (75.5783, 56.3791) (75.6605, 56.543) (75.7421, 56.7075) (75.8231, 56.8725) (75.9034, 57.0379) (75.9831, 57.2039) (76.0622, 57.3704) (76.1407, 57.5373) (76.2185, 57.7047) (76.2957, 57.8726) (76.357, 58.0073) (76.4027, 58.1086) (76.433, 58.1761) (76.4482, 58.21) knots 0 0 0 0 0 0 0.01428571 0.02857143 0.04285714 0.05714286 0.07142857 0.08571429 0.1 0.11428571 0.12857143 0.14285714 0.15714286 0.17142857 0.18571429 0.2 0.21428571 0.22857143 0.24285714 0.25714286 0.27142857 0.28571429 0.3 0.31428571 0.32857143 0.34285714 0.35714286 0.37142857 0.38571429 0.4 0.41428571 0.42857143 0.44285714 0.45714286 0.47142857 0.48571429 0.5 0.51428571 0.52857143 0.54285714 0.55714286 0.57142857 0.58571429 0.6 0.61428571 0.62857143 0.64285714 0.65714286 0.67142857 0.68571429 0.7 0.71428571 0.72857143 0.74285714 0.75714286 0.77142857 0.78571429 0.8 0.81428571 0.82857143 0.84285714 0.85714286 0.87142857 0.88571429 0.9 0.91428571 0.92857143 0.94285714 0.95714286 0.97142857 0.98571429 1 1 1 1 1 1
  arc A66 (76.4482, 58.21) -> (73.5542, 61.8389) centre (0.5538, 0.6546) ccw
  spline S31 degree 5 poles (62.0072, 57.2425) (62.0327, 57.266) (62.0842, 57.3122) (62.163, 57.3797) (62.2711, 57.4659) (62.4104, 57.5687) (62.5526, 57.6679) (62.6966, 57.7648) (62.8416, 57.8605) (62.9873, 57.9555) (63.1336, 58.0495) (63.2808, 58.1424) (63.4292, 58.2337) (63.579, 58.3233) (63.7301, 58.411) (63.8824, 58.4971) (64.0358, 58.5818) (64.1901, 58.6652) (64.3452, 58.7476) (64.5009, 58.829) (64.6573, 58.9094) (64.8144, 58.9887) (64.9723, 59.067) (65.131, 59.144) (65.2905, 59.22) (65.4507, 59.2948) (65.6116, 59.3686) (65.7731, 59.4414) (65.9353, 59.5133) (66.0981, 59.5842) (66.2614, 59.6542) (66.4254, 59.7232) (66.5899, 59.7913) (66.7551, 59.8585) (66.9208, 59.9248) (67.0871, 59.9901) (67.2539, 60.0545) (67.4212, 60.1181) (67.5891, 60.1808) (67.7575, 60.2427) (67.9263, 60.3037) (68.0957, 60.3638) (68.2655, 60.4231) (68.4359, 60.4816) (68.6067, 60.5392) (68.7779, 60.596) (68.9497, 60.652) (69.1218, 60.7072) (69.2944, 60.7616) (69.4675, 60.8152) (69.6409, 60.8681) (69.8148, 60.9201) (69.9891, 60.9713) (70.1639, 61.0218) (70.339, 61.0715) (70.5145, 61.1204) (70.6904, 61.1686) (70.8667, 61.216) (71.0434, 61.2627) (71.2204, 61.3086) (71.3978, 61.3538) (71.5756, 61.3982) (71.7538, 61.4419) (71.9323, 61.4849) (72.1112, 61.5271) (72.2904, 61.5686) (72.4699, 61.6094) (72.6498, 61.6494) (72.83, 61.6888) (73.0105, 61.7274) (73.1914, 61.7653) (73.3364, 61.7951) (73.4452, 61.8171) (73.5179, 61.8316) (73.5542, 61.8389) knots 0 0 0 0 0 0 0.01428571 0.02857143 0.04285714 0.05714286 0.07142857 0.08571429 0.1 0.11428571 0.12857143 0.14285714 0.15714286 0.17142857 0.18571429 0.2 0.21428571 0.22857143 0.24285714 0.25714286 0.27142857 0.28571429 0.3 0.31428571 0.32857143 0.34285714 0.35714286 0.37142857 0.38571429 0.4 0.41428571 0.42857143 0.44285714 0.45714286 0.47142857 0.48571429 0.5 0.51428571 0.52857143 0.54285714 0.55714286 0.57142857 0.58571429 0.6 0.61428571 0.62857143 0.64285714 0.65714286 0.67142857 0.68571429 0.7 0.71428571 0.72857143 0.74285714 0.75714286 0.77142857 0.78571429 0.8 0.81428571 0.82857143 0.84285714 0.85714286 0.87142857 0.88571429 0.9 0.91428571 0.92857143 0.94285714 0.95714286 0.97142857 0.98571429 1 1 1 1 1 1
  line L31 (62.0072, 57.2425) -> (60.9079, 56.2305)
  arc A67 (59.7916, 56.2712) -> (60.9079, 56.2305) centre (60.3703, 56.8145) ccw
  arc A68 (59.7916, 56.2712) -> (56.1704, 59.8924) centre (0.5538, 0.6546) ccw
  arc A69 (56.1297, 61.0086) -> (56.1704, 59.8924) centre (56.7137, 60.4711) ccw
  line L32 (56.1297, 61.0086) -> (57.1417, 62.108)
  spline S32 degree 5 poles (57.1417, 62.108) (57.1652, 62.1335) (57.2114, 62.185) (57.2789, 62.2638) (57.3651, 62.3719) (57.4679, 62.5112) (57.5671, 62.6534) (57.664, 62.7974) (57.7597, 62.9424) (57.8547, 63.0881) (57.9487, 63.2344) (58.0416, 63.3816) (58.1329, 63.53) (58.2225, 63.6797) (58.3102, 63.8309) (58.3963, 63.9832) (58.481, 64.1366) (58.5644, 64.2909) (58.6468, 64.4459) (58.7282, 64.6017) (58.8086, 64.7581) (58.8879, 64.9152) (58.9662, 65.0731) (59.0432, 65.2318) (59.1192, 65.3913) (59.194, 65.5515) (59.2678, 65.7124) (59.3406, 65.8739) (59.4125, 66.0361) (59.4834, 66.1989) (59.5534, 66.3622) (59.6224, 66.5262) (59.6905, 66.6907) (59.7577, 66.8559) (59.824, 67.0216) (59.8893, 67.1879) (59.9537, 67.3547) (60.0173, 67.522) (60.08, 67.6899) (60.1419, 67.8583) (60.2029, 68.0271) (60.263, 68.1965) (60.3223, 68.3663) (60.3808, 68.5367) (60.4384, 68.7075) (60.4952, 68.8787) (60.5512, 69.0505) (60.6064, 69.2226) (60.6608, 69.3952) (60.7144, 69.5683) (60.7673, 69.7417) (60.8193, 69.9156) (60.8705, 70.0899) (60.921, 70.2647) (60.9707, 70.4398) (61.0196, 70.6153) (61.0678, 70.7912) (61.1152, 70.9675) (61.1619, 71.1442) (61.2078, 71.3212) (61.253, 71.4986) (61.2974, 71.6764) (61.3411, 71.8546) (61.3841, 72.0331) (61.4263, 72.212) (61.4678, 72.3912) (61.5086, 72.5707) (61.5486, 72.7506) (61.588, 72.9308) (61.6266, 73.1113) (61.6645, 73.2922) (61.6943, 73.4372) (61.7163, 73.546) (61.7308, 73.6187) (61.7381, 73.655) knots 0 0 0 0 0 0 0.01428571 0.02857143 0.04285714 0.05714286 0.07142857 0.08571429 0.1 0.11428571 0.12857143 0.14285714 0.15714286 0.17142857 0.18571429 0.2 0.21428571 0.22857143 0.24285714 0.25714286 0.27142857 0.28571429 0.3 0.31428571 0.32857143 0.34285714 0.35714286 0.37142857 0.38571429 0.4 0.41428571 0.42857143 0.44285714 0.45714286 0.47142857 0.48571429 0.5 0.51428571 0.52857143 0.54285714 0.55714286 0.57142857 0.58571429 0.6 0.61428571 0.62857143 0.64285714 0.65714286 0.67142857 0.68571429 0.7 0.71428571 0.72857143 0.74285714 0.75714286 0.77142857 0.78571429 0.8 0.81428571 0.82857143 0.84285714 0.85714286 0.87142857 0.88571429 0.9 0.91428571 0.92857143 0.94285714 0.95714286 0.97142857 0.98571429 1 1 1 1 1 1
  arc A70 (61.7381, 73.655) -> (58.1092, 76.549) centre (0.5538, 0.6546) ccw
  spline S33 degree 5 poles (47.8745, 69.4984) (47.8941, 69.527) (47.934, 69.5835) (47.9958, 69.6668) (48.082, 69.7749) (48.1949, 69.9061) (48.3115, 70.0344) (48.4304, 70.161) (48.5504, 70.2866) (48.6713, 70.4116) (48.793, 70.5358) (48.9159, 70.6591) (49.0402, 70.7812) (49.1663, 70.9018) (49.2941, 71.021) (49.4235, 71.1388) (49.5542, 71.2555) (49.6861, 71.3712) (49.8189, 71.486) (49.9526, 71.6) (50.0871, 71.7132) (50.2227, 71.8255) (50.3592, 71.9369) (50.4968, 72.0473) (50.6354, 72.1569) (50.7749, 72.2655) (50.9154, 72.3732) (51.0567, 72.4802) (51.1988, 72.5863) (51.3417, 72.6917) (51.4854, 72.7962) (51.6299, 72.9) (51.7751, 73.0031) (51.9212, 73.1053) (52.068, 73.2068) (52.2156, 73.3075) (52.3638, 73.4074) (52.5129, 73.5066) (52.6626, 73.6051) (52.8129, 73.7029) (52.964, 73.7999) (53.1157, 73.8962) (53.2681, 73.9919) (53.4212, 74.0868) (53.5749, 74.181) (53.7292, 74.2745) (53.8842, 74.3673) (54.0397, 74.4594) (54.1959, 74.5508) (54.3527, 74.6416) (54.51, 74.7317) (54.668, 74.8211) (54.8265, 74.9099) (54.9856, 74.998) (55.1453, 75.0854) (55.3055, 75.1721) (55.4663, 75.2583) (55.6276, 75.3437) (55.7895, 75.4285) (55.9519, 75.5127) (56.1148, 75.5962) (56.2783, 75.6791) (56.4422, 75.7613) (56.6067, 75.8429) (56.7717, 75.9239) (56.9371, 76.0042) (57.1031, 76.0839) (57.2696, 76.163) (57.4365, 76.2415) (57.6039, 76.3193) (57.7718, 76.3965) (57.9065, 76.4578) (58.0078, 76.5035) (58.0753, 76.5338) (58.1092, 76.549) knots 0 0 0 0 0 0 0.01428571 0.02857143 0.04285714 0.05714286 0.07142857 0.08571429 0.1 0.11428571 0.12857143 0.14285714 0.15714286 0.17142857 0.18571429 0.2 0.21428571 0.22857143 0.24285714 0.25714286 0.27142857 0.28571429 0.3 0.31428571 0.32857143 0.34285714 0.35714286 0.37142857 0.38571429 0.4 0.41428571 0.42857143 0.44285714 0.45714286 0.47142857 0.48571429 0.5 0.51428571 0.52857143 0.54285714 0.55714286 0.57142857 0.58571429 0.6 0.61428571 0.62857143 0.64285714 0.65714286 0.67142857 0.68571429 0.7 0.71428571 0.72857143 0.74285714 0.75714286 0.77142857 0.78571429 0.8 0.81428571 0.82857143 0.84285714 0.85714286 0.87142857 0.88571429 0.9 0.91428571 0.92857143 0.94285714 0.95714286 0.97142857 0.98571429 1 1 1 1 1 1
  line L33 (47.8745, 69.4984) -> (47.0279, 68.2671)
  arc A71 (45.9305, 68.0584) -> (47.0279, 68.2671) centre (46.3738, 68.7168) ccw
  arc A72 (45.9305, 68.0584) -> (41.5943, 70.783) centre (0.5538, 0.6546) ccw
  arc A73 (41.3063, 71.8622) -> (41.5943, 70.783) centre (41.9952, 71.4681) ccw
  line L34 (41.3063, 71.8622) -> (42.0483, 73.1593)
  spline S34 degree 5 poles (42.0483, 73.1593) (42.0655, 73.1893) (42.0991, 73.2498) (42.1473, 73.3417) (42.2074, 73.4662) (42.2766, 73.6249) (42.3416, 73.7856) (42.4041, 73.9476) (42.4651, 74.1103) (42.5253, 74.2734) (42.5844, 74.437) (42.6422, 74.6011) (42.6982, 74.7661) (42.7522, 74.9321) (42.8041, 75.0989) (42.8542, 75.2666) (42.9025, 75.435) (42.9496, 75.604) (42.9954, 75.7735) (43.0401, 75.9434) (43.0837, 76.1138) (43.1261, 76.2846) (43.1672, 76.456) (43.207, 76.6278) (43.2456, 76.8002) (43.2829, 76.973) (43.319, 77.1463) (43.354, 77.32) (43.388, 77.4941) (43.4209, 77.6686) (43.4528, 77.8434) (43.4836, 78.0187) (43.5134, 78.1942) (43.5422, 78.3702) (43.5699, 78.5465) (43.5966, 78.7231) (43.6223, 78.9001) (43.6471, 79.0774) (43.6708, 79.255) (43.6937, 79.4329) (43.7155, 79.6111) (43.7365, 79.7896) (43.7565, 79.9684) (43.7756, 80.1475) (43.7938, 80.3268) (43.8111, 80.5064) (43.8275, 80.6863) (43.843, 80.8664) (43.8576, 81.0468) (43.8714, 81.2275) (43.8842, 81.4083) (43.8963, 81.5894) (43.9075, 81.7708) (43.9178, 81.9523) (43.9273, 82.1341) (43.9359, 82.3161) (43.9437, 82.4984) (43.9507, 82.6808) (43.9569, 82.8634) (43.9623, 83.0462) (43.9669, 83.2293) (43.9706, 83.4125) (43.9736, 83.5959) (43.9757, 83.7795) (43.9771, 83.9633) (43.9777, 84.1472) (43.9775, 84.3313) (43.9765, 84.5156) (43.9748, 84.7001) (43.9723, 84.8847) (43.969, 85.0694) (43.9657, 85.2174) (43.963, 85.3284) (43.961, 85.4025) (43.9599, 85.4395) knots 0 0 0 0 0 0 0.01428571 0.02857143 0.04285714 0.05714286 0.07142857 0.08571429 0.1 0.11428571 0.12857143 0.14285714 0.15714286 0.17142857 0.18571429 0.2 0.21428571 0.22857143 0.24285714 0.25714286 0.27142857 0.28571429 0.3 0.31428571 0.32857143 0.34285714 0.35714286 0.37142857 0.38571429 0.4 0.41428571 0.42857143 0.44285714 0.45714286 0.47142857 0.48571429 0.5 0.51428571 0.52857143 0.54285714 0.55714286 0.57142857 0.58571429 0.6 0.61428571 0.62857143 0.64285714 0.65714286 0.67142857 0.68571429 0.7 0.71428571 0.72857143 0.74285714 0.75714286 0.77142857 0.78571429 0.8 0.81428571 0.82857143 0.84285714 0.85714286 0.87142857 0.88571429 0.9 0.91428571 0.92857143 0.94285714 0.95714286 0.97142857 0.98571429 1 1 1 1 1 1
  arc A74 (43.9599, 85.4395) -> (39.7781, 87.4534) centre (0.5538, 0.6546) ccw
  spline S35 degree 5 poles (31.3689, 78.3022) (31.3817, 78.3344) (31.408, 78.3984) (31.4497, 78.4934) (31.5097, 78.618) (31.5906, 78.771) (31.6757, 78.922) (31.7634, 79.0719) (31.8525, 79.221) (31.9425, 79.3697) (32.0336, 79.518) (32.1259, 79.6655) (32.2199, 79.8122) (32.316, 79.9579) (32.4141, 80.1025) (32.514, 80.2462) (32.6155, 80.389) (32.7183, 80.5311) (32.8222, 80.6726) (32.9272, 80.8135) (33.0332, 80.9538) (33.1404, 81.0935) (33.2487, 81.2324) (33.3583, 81.3707) (33.469, 81.5083) (33.5809, 81.6453) (33.6938, 81.7816) (33.8078, 81.9173) (33.9227, 82.0524) (34.0386, 82.1869) (34.1554, 82.3208) (34.2732, 82.4542) (34.3919, 82.587) (34.5115, 82.7191) (34.6321, 82.8507) (34.7535, 82.9817) (34.8758, 83.1122) (34.999, 83.242) (35.1231, 83.3714) (35.2479, 83.5001) (35.3736, 83.6284) (35.5001, 83.756) (35.6274, 83.8832) (35.7555, 84.0098) (35.8844, 84.1358) (36.014, 84.2613) (36.1444, 84.3863) (36.2756, 84.5107) (36.4075, 84.6346) (36.5402, 84.758) (36.6735, 84.8808) (36.8076, 85.0031) (36.9425, 85.1249) (37.078, 85.2462) (37.2142, 85.367) (37.3511, 85.4872) (37.4887, 85.607) (37.6269, 85.7262) (37.7659, 85.8449) (37.9055, 85.9631) (38.0457, 86.0807) (38.1866, 86.1979) (38.3282, 86.3146) (38.4704, 86.4307) (38.6132, 86.5464) (38.7566, 86.6615) (38.9007, 86.7762) (39.0454, 86.8903) (39.1907, 87.0039) (39.3366, 87.1171) (39.4831, 87.2297) (39.6008, 87.3194) (39.6893, 87.3865) (39.7485, 87.4311) (39.7781, 87.4534) knots 0 0 0 0 0 0 0.01428571 0.02857143 0.04285714 0.05714286 0.07142857 0.08571429 0.1 0.11428571 0.12857143 0.14285714 0.15714286 0.17142857 0.18571429 0.2 0.21428571 0.22857143 0.24285714 0.25714286 0.27142857 0.28571429 0.3 0.31428571 0.32857143 0.34285714 0.35714286 0.37142857 0.38571429 0.4 0.41428571 0.42857143 0.44285714 0.45714286 0.47142857 0.48571429 0.5 0.51428571 0.52857143 0.54285714 0.55714286 0.57142857 0.58571429 0.6 0.61428571 0.62857143 0.64285714 0.65714286 0.67142857 0.68571429 0.7 0.71428571 0.72857143 0.74285714 0.75714286 0.77142857 0.78571429 0.8 0.81428571 0.82857143 0.84285714 0.85714286 0.87142857 0.88571429 0.9 0.91428571 0.92857143 0.94285714 0.95714286 0.97142857 0.98571429 1 1 1 1 1 1
  line L35 (31.3689, 78.3022) -> (30.8175, 76.9134)
  arc A75 (29.7941, 76.4657) -> (30.8175, 76.9134) centre (30.0797, 77.2063) ccw
  arc A76 (29.7941, 76.4657) -> (24.9603, 78.1571) centre (0.5538, 0.6546) ccw
  arc A77 (24.4393, 79.1452) -> (24.9603, 78.1571) centre (25.1987, 78.9142) ccw
  line L36 (24.4393, 79.1452) -> (24.8741, 80.5748)